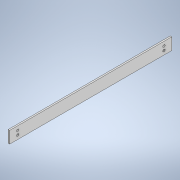
# Autodesk Inventor part: plateHolder2
Saved by Autodesk Inventor 2020 (Build 240168000, 168)
## iProperties
Created: 2019-06-20
Part Number: plateHolder2
Material: Generic
Document SubType Name: Modeling
Designer: Vivek Muskan
Density: 1 g/cm^3
Appearance: Default
Author: Vivek Muskan
Autodesk Inventor part; units mm, degrees
ref_plane "YZ Plane" through (0, 0, 0) normal (1, 0, 0) x (0, 1, 0)
ref_plane "XZ Plane" through (0, 0, 0) normal (0, 1, 0) x (-1, 0, 0)
ref_plane "XY Plane" through (0, 0, 0) normal (0, 0, 1) x (1, 0, 0)
sketch "Sketch1" plane through (0, 0, 0) normal (1, 0, 0) x (0, 1, 0)
  line L0 (0, 0) -> (-15, 0)
  line L1 (-15, 0) -> (-15, -205)
  line L2 (-15, -205) -> (0, -205)
  line L3 (0, -205) -> (0, 0)
  line L4 (-15, -205) -> (-15, -195)
  line L5 (-15, -195) -> (-10, -195)
  circle A0 centre (-10, -195) radius 1.5
  line L6 (-10, -195) -> (-5, -195)
  circle A1 centre (-5, -195) radius 1.5
  line L7 (0, -102.5) -> (-15, -102.5)
  circle A2 centre (-10, -10) radius 1.5
  circle A3 centre (-5, -10) radius 1.5
  dimension "d0" = 15
  dimension "d1" = 205
  dimension "d2" = 10
  dimension "d3" = 5
  dimension "d4" = 3
  dimension "d5" = 5
  dimension "d6" = 3
  constraints: 16 end point, 4 centre point, 3 parallel, 2 coincident, 2 horizontal, 2 midpoint, 2 symmetric about line, 1 perpendicular, 1 point on line, 2 other
  measures "d0" distance of L2.end L1.end
  measures "d1" distance of L1.end L0.end
  measures "d2" distance of L1.end L4.end
  measures "d3" distance of L4.end L5.end
  measures "d4" diameter of A0
  measures "d5" distance of L6.start L6.end
  measures "d6" diameter of A1
extrude "Extrusion1" add sketch "Sketch1" along normal blind 2
body "Solid1"
